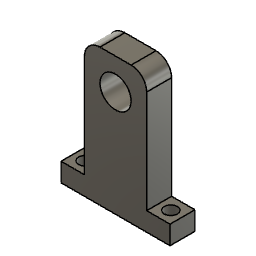
Support tige filetée (Autodesk Fusion 360 design; units mm, degrees)
Autodesk Fusion 360 part; units mm, degrees
sketch "Esquisse1" plane through (0, 0, 0) normal (0, 0, 1) x (1, 0, 0)
  line L0 (0, 0) -> (35, 0)
  line L1 (35, 0) -> (35, 6)
  line L2 (35, 6) -> (0, 6)
  line L3 (0, 6) -> (0, 0)
  line L4 (7.5, 6) -> (27.5, 6)
  line L5 (27.5, 6) -> (27.5, 44)
  line L6 (27.5, 44) -> (7.5, 44)
  line L7 (7.5, 44) -> (7.5, 6)
  circle A0 centre (17.5, 34) radius 5
  line L8 (7.5, 44) -> (27.5, 44) construction
  line L9 (27.5, 44) -> (27.5, 24) construction
  line L10 (27.5, 24) -> (7.5, 24) construction
  line L11 (7.5, 24) -> (7.5, 44) construction
  line L12 (7.5, 44) -> (27.5, 24) construction
  line L13 (27.5, 44) -> (7.5, 24) construction
  dimension "d1" = 35
  dimension "d2" = 6
  dimension "d3" = 20
  dimension "d5" = 10
  dimension "d6" = 20
  dimension "d7" = 20
  dimension "d10" = 34
  constraint horizontal L0
  constraint vertical L1
  constraint horizontal L2
  constraint vertical L3
  constraint coincident L0.start L3.end
  constraint horizontal L4
  constraint vertical L5
  constraint horizontal L6
  constraint vertical L7
  constraint coincident L2 L4.start
  constraint midpoint L2 L4
  constraint horizontal L8
  constraint vertical L9
  constraint horizontal L10
  constraint vertical L11
  constraint midpoint A0.centre L13
  measures "d1" distance of L0.start L0.end
  measures "d2" distance of L0.start L2.end
  measures "d3" distance of L4.start L4.end
  measures "d5" diameter of A0
  measures "d6" distance of L6.end L5.end
  measures "d7" distance of L6.end L10.end
  measures "d10" distance of L0 A0.centre
extrude "Extrusion1" add sketch "Esquisse1" along normal blind 8
sketch "Esquisse2" plane through (0, 6, 0) normal (0, 1, 0) x (-1, 0, 0)
  line L0 (-7.5, 0) -> (0, 0)
  line L1 (0, 0) -> (0, 8)
  line L2 (0, 8) -> (-7.5, 8)
  line L3 (-7.5, 8) -> (-7.5, 0)
  circle A0 centre (-3.75, 4) radius 2.1
  line L4 (0, 0) -> (-7.5, 8) construction
  line L5 (-7.5, 0) -> (0, 8) construction
  dimension "d11" = 4.2
  constraint coincident L0.end L1.start
  constraint coincident L2.end L3.start
  constraint coincident L0.start L3.end
  constraint coincident L1.end L2.start
  constraint midpoint A0.centre L5
  measures "d11" diameter of A0
sketch "Esquisse3" plane through (0, 6, 0) normal (0, 1, 0) x (-1, 0, 0)
  line L0 (-35, 0) -> (-27.5, 0)
  line L1 (-27.5, 0) -> (-27.5, 8)
  line L2 (-27.5, 8) -> (-35, 8)
  line L3 (-35, 8) -> (-35, 0)
  line L4 (-27.5, 0) -> (-35, 8) construction
  line L5 (-35, 0) -> (-27.5, 8) construction
  circle A0 centre (-31.25, 4) radius 2.1
  dimension "d12" = 4.2
  constraint coincident L0.end L1.start
  constraint coincident L2.end L3.start
  constraint coincident L0.start L3.end
  constraint coincident L1.end L2.start
  constraint midpoint L4 A0.centre
  measures "d12" diameter of A0
extrude "Extrusion2" cut sketch "Esquisse2" sketch "Esquisse3" against normal blind 10 contours A0 of sketch 2 contours A0
fillet "Congé1" radius 0.5 2 edges at (5.7079, 0, 3.2406) (33.2079, 0, 3.2406)
fillet "Congé2" radius 5 2 edges at (7.5, 44, 4) (27.5, 44, 4)
